Autodesk Fusion 360 part; units mm, degrees
(part 4 of 4)
sketch "Sketch2" plane through (0, 0, 0) normal (0, 1, 0) x (-1, 0, 0)
  line L0 (13, -8.25) -> (13, -4.1)
  line L1 (13, -4.1) -> (14, -4.1)
  line L2 (13, -4.1) -> (14, -4.1)
  line L3 (14, -4.1) -> (14, -5.1)
  line L4 (14, -5.1) -> (15, -5.1)
  line L5 (15, -5.1) -> (15, -13)
  line L6 (5.1, -15) -> (13, -15)
  line L7 (13, -15) -> (5.1, -15)
  line L8 (5.1, -14) -> (4.1, -14)
  line L9 (4.1, -14) -> (4.1, -13)
  line L10 (4.1, -13) -> (8.25, -13)
  arc A0 (13, -15) -> (15, -13) centre (13, -13) ccw
  line L11 (12.5, -13.5) -> (10.75, -13.5)
  line L12 (9.75, -12.5) -> (9.75, -10.75)
  line L13 (10.75, -9.75) -> (12.5, -9.75)
  line L14 (13.5, -10.75) -> (13.5, -12.5)
  arc A1 (12.5, -13.5) -> (13.5, -12.5) centre (12.5, -12.5) ccw
  line L15 (12.5, -12.5) -> (-13, 13)
  arc A2 (12.5, -13.5) -> (13.5, -12.5) centre (12.5, -12.5) ccw
  arc A3 (9.75, -12.5) -> (10.75, -13.5) centre (10.75, -12.5) ccw
  arc A4 (10.75, -9.75) -> (9.75, -10.75) centre (10.75, -10.75) ccw
  arc A5 (13.5, -10.75) -> (12.5, -9.75) centre (12.5, -10.75) ccw
  line L16 (15, -13) -> (15, -5.1)
  line L17 (12.5, -9.75) -> (10.75, -9.75)
  line L18 (10.75, -13.5) -> (12.5, -13.5)
  line L19 (9.5009, -9.5009) -> (1.6153, -1.6153) construction
  line L20 (8.25, -13) -> (8.25, -9.6642)
  line L21 (8.25, -10.6606) -> (8.25, -13)
  line L22 (13, -8.25) -> (9.6642, -8.25)
  line L23 (5.1, -14) -> (5.1, -15)
  line L24 (9.6642, -8.25) -> (5.5142, -4.1)
  line L25 (8.25, -9.6642) -> (4.1, -5.5142)
  line L26 (13.5, 10.75) -> (13.5, 12.5)
  arc A6 (13.5, 12.5) -> (12.5, 13.5) centre (12.5, 12.5) ccw
  arc A7 (10.75, 13.5) -> (9.75, 12.5) centre (10.75, 12.5) ccw
  line L27 (9.75, 12.5) -> (9.75, 10.75)
  line L28 (9.5009, 9.5009) -> (1.6153, 1.6153) construction
  line L29 (13, 8.25) -> (13, 4.1)
  arc A8 (9.75, 10.75) -> (10.75, 9.75) centre (10.75, 10.75) ccw
  line L30 (13, 4.1) -> (14, 4.1)
  arc A9 (13.5, 12.5) -> (12.5, 13.5) centre (12.5, 12.5) ccw
  line L31 (13, 4.1) -> (14, 4.1)
  line L32 (14, 4.1) -> (14, 5.1)
  line L33 (14, 5.1) -> (15, 5.1)
  line L34 (10.75, 9.75) -> (12.5, 9.75)
  line L35 (12.5, 9.75) -> (10.75, 9.75)
  line L36 (13, 8.25) -> (9.6642, 8.25)
  arc A10 (12.5, 9.75) -> (13.5, 10.75) centre (12.5, 10.75) ccw
  line L37 (4.1, 14) -> (4.1, 13)
  line L38 (5.1, 14) -> (4.1, 14)
  line L39 (15, 13) -> (15, 5.1)
  line L40 (15, 5.1) -> (15, 13)
  line L41 (5.1, 15) -> (13, 15)
  line L42 (13, 15) -> (5.1, 15)
  line L43 (4.1, 13) -> (8.25, 13)
  line L44 (12.5, 13.5) -> (10.75, 13.5)
  line L45 (10.75, 13.5) -> (12.5, 13.5)
  line L46 (8.25, 13) -> (8.25, 9.6642)
  line L47 (9.6642, 8.25) -> (5.5142, 4.1)
  line L48 (8.25, 10.6606) -> (8.25, 13)
  arc A11 (15, 13) -> (13, 15) centre (13, 13) ccw
  line L49 (8.25, 9.6642) -> (4.1, 5.5142)
  line L50 (5.1, 14) -> (5.1, 15)
  line L51 (-8.25, 9.6642) -> (-4.1, 5.5142)
  line L52 (-8.25, 10.6606) -> (-8.25, 13)
  line L53 (-12.5, -13.5) -> (-10.75, -13.5)
  arc A12 (-10.75, 9.75) -> (-9.75, 10.75) centre (-10.75, 10.75) ccw
  line L54 (-8.25, 13) -> (-8.25, 9.6642)
  line L55 (-4.1, -13) -> (-8.25, -13)
  line L56 (-15, -5.1) -> (-15, -13)
  line L57 (-9.75, 12.5) -> (-9.75, 10.75)
  line L58 (-13, -8.25) -> (-13, -4.1)
  line L59 (-8.25, -10.6606) -> (-8.25, -13)
  line L60 (-13, 8.25) -> (-13, 4.1)
  line L61 (-12.5, 13.5) -> (-10.75, 13.5)
  line L62 (-4.1, 13) -> (-8.25, 13)
  line L63 (-4.1, -14) -> (-4.1, -13)
  line L64 (-13, -15) -> (-5.1, -15)
  line L65 (-13.5, 10.75) -> (-13.5, 12.5)
  line L66 (-8.25, -13) -> (-8.25, -9.6642)
  line L67 (-9.6642, 8.25) -> (-5.5142, 4.1)
  arc A13 (-12.5, 13.5) -> (-13.5, 12.5) centre (-12.5, 12.5) ccw
  line L68 (-10.75, 13.5) -> (-12.5, 13.5)
  arc A14 (-13.5, -12.5) -> (-12.5, -13.5) centre (-12.5, -12.5) ccw
  line L69 (-13, -8.25) -> (-9.6642, -8.25)
  arc A15 (-12.5, -9.75) -> (-13.5, -10.75) centre (-12.5, -10.75) ccw
  arc A16 (-10.75, -13.5) -> (-9.75, -12.5) centre (-10.75, -12.5) ccw
  line L70 (-14, 5.1) -> (-15, 5.1)
  line L71 (-14, -5.1) -> (-15, -5.1)
  line L72 (-13, 15) -> (-5.1, 15)
  line L73 (-10.75, 9.75) -> (-12.5, 9.75)
  line L74 (-13, -4.1) -> (-14, -4.1)
  line L75 (-5.1, -14) -> (-5.1, -15)
  line L76 (-14, 4.1) -> (-14, 5.1)
  arc A17 (-9.75, -10.75) -> (-10.75, -9.75) centre (-10.75, -10.75) ccw
  line L77 (-14, -4.1) -> (-14, -5.1)
  line L78 (-15, 13) -> (-15, 5.1)
  line L79 (-10.75, -13.5) -> (-12.5, -13.5)
  line L80 (-13.5, -10.75) -> (-13.5, -12.5)
  line L81 (-5.1, -15) -> (-13, -15)
  arc A18 (-9.75, 12.5) -> (-10.75, 13.5) centre (-10.75, 12.5) ccw
  line L82 (-13, 4.1) -> (-14, 4.1)
  line L83 (-13, -4.1) -> (-14, -4.1)
  line L84 (-5.1, 14) -> (-5.1, 15)
  line L85 (-8.25, -9.6642) -> (-4.1, -5.5142)
  line L86 (-13, 4.1) -> (-14, 4.1)
  arc A19 (-13.5, 10.75) -> (-12.5, 9.75) centre (-12.5, 10.75) ccw
  line L87 (-15, -13) -> (-15, -5.1)
  line L88 (-9.5009, 9.5009) -> (-1.6152, 1.6153) construction
  line L89 (-10.75, -9.75) -> (-12.5, -9.75)
  line L90 (-5.1, 14) -> (-4.1, 14)
  line L91 (-15, 5.1) -> (-15, 13)
  line L92 (-9.75, -12.5) -> (-9.75, -10.75)
  arc A20 (-13, 15) -> (-15, 13) centre (-13, 13) ccw
  line L93 (-12.5, -9.75) -> (-10.75, -9.75)
  arc A21 (-15, -13) -> (-13, -15) centre (-13, -13) ccw
  arc A22 (-13.5, -12.5) -> (-12.5, -13.5) centre (-12.5, -12.5) ccw
  arc A23 (-12.5, 13.5) -> (-13.5, 12.5) centre (-12.5, 12.5) ccw
  line L94 (-5.1, -14) -> (-4.1, -14)
  line L95 (-12.5, 9.75) -> (-10.75, 9.75)
  line L96 (-9.5009, -9.5009) -> (-1.6152, -1.6153) construction
  line L97 (-5.1, 15) -> (-13, 15)
  line L98 (-13, 8.25) -> (-9.6642, 8.25)
  line L99 (-9.6642, -8.25) -> (-5.5142, -4.1)
  line L100 (-4.1, 14) -> (-4.1, 13)
  line L101 (4.1, -5.5142) -> (-4.1, -5.5142)
  line L102 (5.5142, 4.1) -> (5.5142, -4.1)
  line L103 (-5.5142, 4.1) -> (-5.5142, -4.1)
  line L104 (4.1, 5.5142) -> (-4.1, 5.5142)
  circle A24 centre (0, 0) radius 3.4
  point P0 (13, -8.25)
  point P1 (14, -4.1)
  point P2 (14, -5.1)
  point P3 (15, -5.1)
  point P4 (15, -15)
  point P5 (5.1, -15)
  point P6 (5.1, -14)
  point P7 (4.1, -14)
  point P8 (4.1, -13)
  point P9 (8.25, -13)
  point P10 (0, 0)
  point P11 (15, 0)
  point P12 (0, 15)
  point P13 (0, 0)
  point P14 (15, 15)
  point P15 (12.5, 12.5)
  point P16 (5.1, 14)
  point P17 (5.1, 15)
  point P18 (8.25, 13)
  point P19 (4.1, 13)
  point P20 (14, 5.1)
  point P21 (4.1, 14)
  point P22 (14, 4.1)
  point P23 (13, 8.25)
  point P24 (15, 5.1)
  point P25 (-12.5, 12.5)
  point P26 (-15, 0)
  point P27 (-5.1, 15)
  point P28 (-8.25, 13)
  point P29 (-4.1, 13)
  point P30 (-5.1, -15)
  point P31 (-15, 15)
  point P32 (-14, 5.1)
  point P33 (-4.1, 14)
  point P34 (-14, 4.1)
  point P35 (-13, 8.25)
  point P36 (-15, 5.1)
  point P37 (-4.1, -13)
  point P38 (0, 0)
  point P39 (0, 0)
  point P40 (0, 15)
  point P41 (0, 15)
  point P42 (0, -15)
  point P43 (0, 0)
  point P44 (-8.25, -13)
  point P45 (-4.1, -14)
  point P46 (-15, -15)
  point P47 (-5.1, -14)
  point P48 (-12.5, -12.5)
  point P49 (0, 0)
  point P50 (-5.1, 14)
  point P51 (-15, -5.1)
  point P52 (-14, -5.1)
  point P53 (-13, -8.25)
  point P54 (-14, -4.1)
  point P55 (-15, 0)
  dimension "d78" = 2
  dimension "d79" = 1
  dimension "d80" = 1.5
  dimension "d91" = 1
  dimension "d92" = 1
  dimension "d93" = 1.5
  dimension "d94" = 1.5
  dimension "d102" = 3.75
  dimension "d103" = 1.5
  dimension "d104" = 3.75
  dimension "d105" = 2
  dimension "d106" = 2
  dimension "d109" = 5.869
  dimension "d110" = 5.869
  dimension "d111" = 3.3358
  dimension "d112" = 3.3358
  dimension "d113" = 4.15
  dimension "d114" = 4.15
  dimension "d115" = 8.2
  dimension "d116" = 8.2
  dimension "d117" = 8.2
  dimension "d118" = 8.2
  dimension "d119" = 6.8
  constraint coincident L0.end L1.start
  constraint coincident P1 L1.end
  constraint coincident P2 L3.end
  constraint coincident P3 L4.end
  constraint coincident P5 L6.start
  constraint coincident P6 L8.start
  constraint coincident P7 L8.end
  constraint coincident P8 L9.end
  constraint coincident P9 L10.end
  constraint tangent L5 A0
  constraint tangent L7 A0
  constraint horizontal L11
  constraint vertical L12
  constraint horizontal L13
  constraint vertical L14
  constraint tangent L14 A2
  constraint tangent L11 A2
  constraint tangent L11 A3
  constraint tangent L12 A3
  constraint equal A2 A3
  constraint tangent L12 A4
  constraint tangent L13 A4
  constraint equal A2 A4
  constraint tangent L13 A5
  constraint tangent L14 A5
  constraint equal A2 A5
  constraint coincident L15 L19.start
  constraint coincident L15 L19.end
  constraint parallel L15 L19
  constraint perpendicular L10 L20
  constraint coincident P0 L0.start
  constraint perpendicular L0 L22
  constraint parallel L19 L24
  constraint parallel L19 L25
  constraint perpendicular L7 L23
  constraint coincident P49 P43
  measures "d78" radius of A0
  measures "d79" radius of A2
  measures "d80" distance of L14 L16
  measures "d91" distance of L19 L24
  measures "d92" distance of L15 L25
  measures "d93" distance of L12 L20
  measures "d94" distance of L13 L22
  measures "d102" distance of L12 L14
  measures "d103" distance of L7 L11
  measures "d104" distance of L11 L13
  measures "d105" distance of L7 L10
  measures "d106" distance of L0 L5
  measures "d109" distance of L22.end L24.end
  measures "d110" distance of L20.end L25.end
  measures "d111" distance of P9 L20.end
  measures "d112" distance of P0 L22.end
  measures "d113" distance of P8 P9
  measures "d114" distance of P0 L0.end
  measures "d115" distance of L25.end L85.end
  measures "d116" distance of L24.end L47.end
  measures "d117" distance of L67.end L99.end
  measures "d118" distance of L49.end L51.end
  measures "d119" diameter of A24
extrude "Extrude1" add sketch "Sketch2" along normal blind 230
move_body "Move1" bodies 1 to x (0, -1, 0) y (1, 0, 0) z (0, 0, 1) at (-3.4, 15.1, 15)
move_body "Move2" bodies 1 to x (1, 0, 0) y (0, 1, 0) z (0, 0, 1) at (3.4, 0, 0)
equation "d33 = ( 8.2 / 2 ) * 1 mm"
equation "d59 = ( 8.5 / 2 ) * 1 mm"
equation "d60 = ( 8.5 / 2 ) * 1 mm"
equation "d72 = ( 8.2 / 2 ) * 1 mm"
equation "Length = 230 mm"

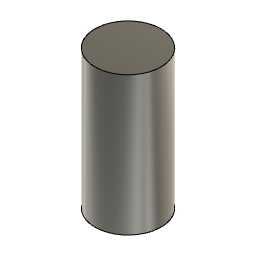
design "differential_joint"
Autodesk Fusion 360 part; units mm, degrees
sketch "Sketch1" plane through (0, 0, 0) normal (0, 0, 1) x (1, 0, 0)
  circle A0 centre (0, 0) radius 8.325
  dimension "d1" = 16.65
  constraint coincident A0.centre origin
  measures "d1" diameter of A0
extrude "Extrude1" add sketch "Sketch1" along normal blind 35
equation "d1 = ( 8.325 * 2 ) * 1 mm"

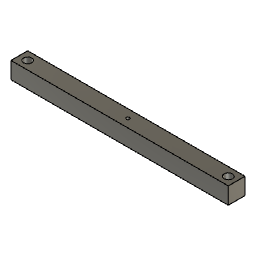
design "differential_bar"
Autodesk Fusion 360 part; units mm, degrees
sketch "Sketch1" plane through (0, 0, 0) normal (0, 0, 1) x (1, 0, 0)
  line L0 (-130, 10) -> (130, 10)
  line L1 (130, 10) -> (130, -10)
  line L2 (130, -10) -> (-130, -10)
  line L3 (-130, -10) -> (-130, 10)
  dimension "d1" = 20
  dimension "d2" = 260
  constraint horizontal L0
  constraint vertical L1
  constraint horizontal L2
  constraint vertical L3
  measures "d1" distance of L0.start L2.end
  measures "d2" distance of L0.start L0.end
sketch "Sketch2" plane through (0, 0, 0) normal (0, 0, 1) x (1, 0, 0)
  circle A0 centre (0, 0) radius 8.325
  dimension "d3" = 16.65
  constraint coincident A0.centre origin
  measures "d3" diameter of A0
extrude "Extrude1" add sketch "Sketch1" along normal blind 20
extrude "Extrude2" cut sketch "Sketch2" along normal blind 10
sketch "Sketch3" plane through (0, 0, 0) normal (0, 0, 1) x (1, 0, 0)
  circle A0 centre (0, 0) radius 2
  dimension "d8" = 4
  constraint coincident A0.centre origin
  measures "d8" diameter of A0
extrude "Extrude3" cut sketch "Sketch3" along normal blind 50
sketch "Sketch4" plane through (0, 0, 20) normal (0, 0, 1) x (-1, 0, 0)
  circle A0 centre (0, 0) radius 2
  line L0 (130, 10) -> (-130, 10)
  line L1 (-130, 10) -> (-130, -10)
  line L2 (-130, -10) -> (130, -10)
  line L3 (130, -10) -> (130, 10)
  circle A1 centre (120, 0) radius 5
  circle A2 centre (-120, 0) radius 5
  dimension "d11" = 10
  dimension "d12" = 10
  measures "d11" diameter of A1
  measures "d12" diameter of A2
extrude "Extrude4" cut sketch "Sketch4" against normal blind 10 contours A1 | A2
sketch "Sketch5" plane through (0, 0, 20) normal (0, 0, 1) x (-1, 0, 0)
  circle A0 centre (120, 0) radius 5
  circle A1 centre (-120, 0) radius 5
  circle A2 centre (0, 0) radius 2
  line L0 (130, 10) -> (-130, 10)
  line L1 (-130, 10) -> (-130, -10)
  line L2 (-130, -10) -> (130, -10)
  line L3 (130, -10) -> (130, 10)
  circle A3 centre (120, 0) radius 2
  circle A4 centre (-120, 0) radius 2
  dimension "d15" = 4
  dimension "d16" = 4
  constraint concentric A0 A3
  constraint concentric A1 A4
  measures "d15" diameter of A3
  measures "d16" diameter of A4
extrude "Extrude5" cut sketch "Sketch5" against normal blind 80 contours A3 | A4
move_body "Move1" bodies 1 to x (1, 0, 0) y (0, 1, 0) z (0, 0, 1) at (0, 0, -10)
equation "d3 = ( 8.325 * 2 ) * 1 mm"
